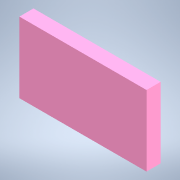
# Autodesk Inventor part: Aduino
Saved by Autodesk Inventor 2022.3 (Build 263350000, 350)
## iProperties
Created: 2023-02-06
Part Number: Aduino
Material: Generic
Document SubType Name: Modeling
Designer: lbmcgill42
Density: 1 g/cm^3
Appearance: Default
Author: lbmcgill42
Autodesk Inventor part; units mm, degrees
ref_plane "YZ Plane" through (0, 0, 0) normal (1, 0, 0) x (0, 1, 0)
ref_plane "XZ Plane" through (0, 0, 0) normal (0, 1, 0) x (-1, 0, 0)
ref_plane "XY Plane" through (0, 0, 0) normal (0, 0, 1) x (1, 0, 0)
sketch "Sketch1" plane through (0, 0, 0) normal (0, 1, 0) x (-1, 0, 0)
  line L0 (3.8717, 4.9034) -> (-110.4283, 4.9034)
  line L1 (-110.4283, 4.9034) -> (-110.4283, -7.7966)
  line L2 (-110.4283, -7.7966) -> (3.8717, -7.7966)
  line L3 (3.8717, -7.7966) -> (3.8717, 4.9034)
  point P0 (0, 0)
  dimension "d0" = 12.7
  dimension "d1" = 114.3
  constraints: 8 end point, 2 parallel, 1 horizontal, 1 perpendicular
  measures "d0" distance of L2.end L0.start
  measures "d1" distance of L0.start L0.end
extrude "Extrusion1" add sketch "Sketch1" along normal blind 63.5
body "Solid1"
